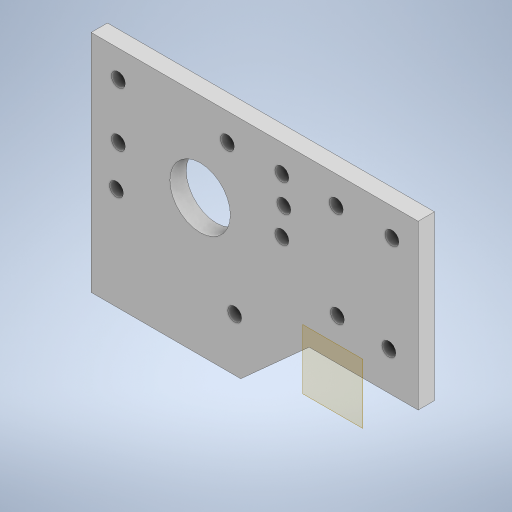
# Autodesk Inventor part: Y axis motor mount new
Saved by Autodesk Inventor 2023.2 (Build 272271000, 271)
## iProperties
Created: 2023-03-31
Part Number: Y axis motor mount new
Material: Generic
Document SubType Name: Modeling
Designer: dmargari
Density: 1 g/cm^3
Appearance: Default
Author: dmargari
## iProperties of the stored document Y axis motor mount new_3DPrint.ipt
Created: 2023-03-31
Part Number: Y axis motor mount new_3DPrint
Material: Generic
Document SubType Name: Modeling
Designer: dmargari
Density: 1 g/cm^3
Appearance: Default
Author: dmargari
Autodesk Inventor part; units mm, degrees
ref_plane "YZ Plane" through (0, 0, 0) normal (1, 0, 0) x (0, 1, 0)
ref_plane "XZ Plane" through (0, 0, 0) normal (0, 1, 0) x (-1, 0, 0)
ref_plane "XY Plane" through (0, 0, 0) normal (0, 0, 1) x (1, 0, 0)
sketch "Sketch1" plane through (0, 0, 0) normal (0, 0, 1) x (1, 0, 0)
  circle A0 centre (-83.65, 30) radius 2.1 projected
  circle A1 centre (-23.65, 30) radius 2.1 projected
  circle A2 centre (-23.65, 50) radius 2.1 projected
  circle A3 centre (-83.65, 50) radius 2.1 projected
  line L0 (-3.55, 0) -> (-3.5497, 1000) projected
  line L1 (16.25, 0) -> (16.2503, 1000) projected
  line L2 (-93.65, 20.5) -> (-93.65, 25.1685) projected
  line L3 (-73.65, 25.1685) -> (-73.65, 20.5) projected
  line L4 (-78.75, 60) -> (-68.55, 60) projected
  line L5 (-88.55, 20) -> (-93.15, 20) projected
  line L6 (-93.65, 20) -> (-93.65, 60)
  line L7 (-93.65, 60) -> (26.35, 60)
  line L8 (26.35, 60) -> (26.35, 0)
  line L9 (26.35, 0) -> (-3.55, 0)
  line L10 (-93.65, -22.5923) -> (-93.65, 20)
  line L11 (-74.15, 20) -> (-78.75, 20) construction
  line L12 (-33.65, 20.5) -> (-33.65, 25.1685) projected
  line L13 (-53.65, -43.196) -> (-53.65, 110.7641) construction
  line L14 (-13.65, 0) -> (-38.74, -22.5923)
  circle A4 centre (-53.65, 27.5) radius 11.1
  circle A5 centre (-43.65, 50) radius 2.1 projected
  line L15 (-93.65, -22.5923) -> (-38.74, -22.5923)
  line L16 (-13.65, 0) -> (-3.55, 0)
  point P0 (0, 0)
  point P1 (-62.8644, -22.5923)
  point P2 (-93.65, -24.4136)
  point P3 (-3.55, 15)
  point P4 (-3.55, 50)
  point P5 (16.25, 50)
  point P6 (16.25, 15)
  dimension "d0" = 120
  dimension "d1" = 40
  dimension "d5" = 20
  dimension "d36" = 22.2
  dimension "d37" = 32.5
  dimension "d45" = 15
  dimension "d47" = 50
  dimension "d48" = 50
  dimension "d79" = 15
  constraints: 18 end point, 5 point on line, 3 coincident, 2 parallel, 2 perpendicular, 2 vertical, 1 centre point, 1 collinear, 1 horizontal
  measures "d0" distance of L6.end L7.end
  measures "d1" distance of L8.end L14.start
  measures "d5" distance between parallel lines of L3 L13
  measures "d36" diameter of A4
  measures "d37" distance from line of L7 point (-53.65, 27.5)
  measures "d45" distance from line of L9 point (16.25, 15)
  measures "d47" distance from line of L9 point (16.25, 50)
  measures "d48" distance from line of L9 point (-3.55, 50)
  measures "d79" distance from line of L9 point (-3.55, 15)
extrude "Extrusion2" add sketch "Sketch1" against normal blind 6 contours A0 | A1 | A2 | A3 | L16 L14 L15 L10 L6 L2 L7 L4 L0 | L0 L7 L1 L9 | L1 L7 L8 L9 | A5
ref_plane "Work Plane1" through (0, 0, 5) normal (0, 0, 1) x (1, 0, 0)
sketch "Sketch2" plane through (0, 0, 5) normal (0, 0, 1) x (1, 0, 0)
  line L0 (-66.3198, 58.2348) -> (-84.359, 14.8345) construction
  line L1 (-84.359, 14.8345) -> (-40.9587, -3.2047) construction
  line L2 (-40.9587, -3.2047) -> (-22.9195, 40.1957) construction
  line L3 (-22.9195, 40.1957) -> (-66.3198, 58.2348) construction
  line L4 (-66.3198, 58.2348) -> (-40.9587, -3.2047) construction
  line L5 (-84.359, 14.8345) -> (-22.9195, 40.1957) construction
  circle A0 centre (-22.9195, 40.1957) radius 4.6 construction
  circle A1 centre (-84.359, 14.8345) radius 4.6 construction
  point P0 (0, 0)
  point P1 (-53.6392, 27.5151)
  dimension "d41" = 47
  dimension "d42" = 47
  dimension "d43" = 9.2
  dimension "d44" = 9.2
  constraints: 12 end point, 6 coincident, 2 centre point, 2 parallel, 1 midpoint, 1 perpendicular
  measures "d41" distance of L2.end L2.start
  measures "d42" distance of L2.start L0.end
  measures "d43" diameter of A0
  measures "d44" diameter of A1
hole "Hole2" at (-84.359, 14.8345, 5) at (-22.9195, 40.1957, 5) at (-40.9587, -3.2047, 5) direction (0, 0, -1) diameter 5.1 end through all
hole "Hole3" at (-53.65, 27.5, 0) at (-43.65, 50, 0) at (-23.65, 50, 0) at (-23.65, 30, 0) at (-83.65, 50, 0) at (-83.65, 30, 0) direction (0, 0, -1) diameter 5.1 end through all
sketch "Sketch3" plane through (0, 0, 0) normal (0, 0, 1) x (1, 0, 0)
  point P0 (0, 0)
  point P1 (-3.2825, 15.0941)
  point P2 (-3.7043, 49.839)
  point P3 (16.7382, 49.8563)
  point P4 (15.6257, 14.0035)
hole "Hole4" at (-3.2825, 15.0941, 0) at (-3.7043, 49.839, 0) at (16.7382, 49.8563, 0) at (15.6257, 14.0035, 0) direction (0, 0, -1) diameter 5.1 end through all
body "Solid2"
